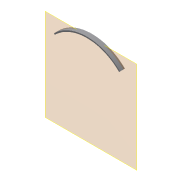
# Autodesk Inventor part: Cover
Saved by Autodesk Inventor 2017 (Build 210142000, 142)
## iProperties
Created: 2017-03-15
Part Number: Cover
Material: Generic
Document SubType Name: Modeling
Designer: zallen
Density: 1 g/cm^3
Appearance: Default
Author: zallen
Autodesk Inventor part; units mm, degrees
ref_plane "YZ Plane" through (0, 0, 0) normal (1, 0, 0) x (0, 1, 0)
ref_plane "XZ Plane" through (0, 0, 0) normal (0, 1, 0) x (-1, 0, 0)
ref_plane "XY Plane" through (0, 0, 0) normal (0, 0, 1) x (1, 0, 0)
sketch "Sketch1" plane through (0, 0, 0) normal (0, 0, 1) x (1, 0, 0)
  line L0 (0, 0) -> (234.95, 0) construction
  line L1 (0, 0) -> (234.95, 0) construction
  line L2 (166.1347, 166.1347) -> (161.6446, 161.6446)
  line L3 (-166.1347, 166.1347) -> (-161.6446, 161.6446)
  arc A0 (161.6446, 161.6446) -> (-161.6446, 161.6446) centre (0, 0) ccw
  arc A1 (166.1347, 166.1347) -> (-166.1347, 166.1347) centre (0, 0) ccw
  line L4 (-166.1347, 166.1347) -> (-170.6249, 170.6249)
  line L5 (166.1347, 166.1347) -> (170.6249, 170.6249)
  arc A2 (170.6249, 170.6249) -> (-170.6249, 170.6249) centre (0, 0) ccw
  dimension "d3" = 234.95
  dimension "d6" = 228.6
  dimension "d9" = 6.35
  dimension "d10" = 6.35
  dimension "d11" = 241.3
  constraints: 12 end point, 6 point on circle, 3 centre point, 2 horizontal, 1 coincident, 1 concentric, 1 point on line
  measures "d3" distance of L0.start L3.start
  measures "d6" radius of A0
  measures "d9" distance of L3.start L4.end
  measures "d10" distance of L2.start L5.end
  measures "d11" radius of A2
extrude "Extrusion2" add sketch "Sketch1" along normal blind 25.4 contours A1 L4 A2 L5
body "Solid2"
